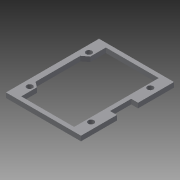
# Autodesk Inventor part: battery_mount
Saved by Autodesk Inventor 2013 (Build 170138000, 138)
## iProperties
Created: 2014-05-23
Part Number: battery_mount
Material: Generic
Document SubType Name: Modeling
Designer: balogh
Density: 1 g/cm^3
Author: balogh
Autodesk Inventor part; units mm, degrees
ref_plane "YZ Plane" through (0, 0, 0) normal (1, 0, 0) x (0, 1, 0)
ref_plane "XZ Plane" through (0, 0, 0) normal (0, 1, 0) x (-1, 0, 0)
ref_plane "XY Plane" through (0, 0, 0) normal (0, 0, 1) x (1, 0, 0)
sketch "Sketch1" plane through (0, 0, 0) normal (0, 0, 1) x (1, 0, 0)
  circle A0 centre (-17.78, 18.415) radius 1.7525
  circle A1 centre (17.7801, 18.4151) radius 1.7525
  circle A2 centre (-17.78, -18.4151) radius 1.7525
  circle A3 centre (17.7799, -18.415) radius 1.7525
  line L0 (6.35, -18.415) -> (-6.35, -18.415)
  line L1 (-6.35, -18.415) -> (-6.35, -22.5171)
  line L2 (-6.35, -22.5171) -> (-27.94, -22.5171)
  line L3 (-27.94, -22.5171) -> (-27.94, 22.513)
  line L4 (-27.94, 22.513) -> (27.94, 22.513)
  line L5 (27.94, 22.513) -> (27.94, -22.5171)
  line L6 (27.94, -22.5171) -> (6.35, -22.5171)
  line L7 (6.35, -22.5171) -> (6.35, -18.415)
  line L8 (16.0276, 15.875) -> (25.4, 15.875)
  line L9 (25.4, 15.875) -> (25.4, -15.875)
  line L10 (25.4, -15.875) -> (-25.4, -15.875)
  line L11 (-25.4, -15.875) -> (-25.4, 15.875)
  line L12 (-25.4, 15.875) -> (-16.0274, 15.875)
  line L13 (-16.0274, 15.875) -> (-13.4874, 19.194)
  line L14 (-13.4874, 19.194) -> (13.4876, 19.194)
  line L15 (13.4876, 19.194) -> (16.0276, 15.875)
  point P0 (0, 0)
  constraints: 32 end point, 6 parallel, 6 perpendicular, 4 centre point, 3 equal radius, 1 collinear
extrude "Extrusion1" add sketch "Sketch1" along normal blind 2.8956
body "Solid1"
